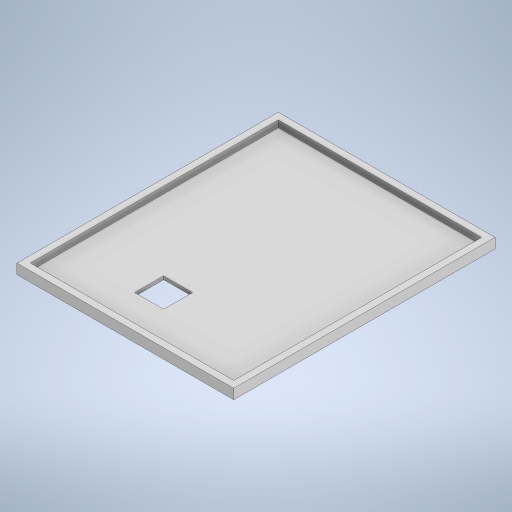
# Autodesk Inventor part: Tampa
Saved by Autodesk Inventor 2024 (Build 280153000, 153)
## iProperties
Created: 2023-09-01
Part Number: Tampa
Material: Genérico
Document SubType Name: Modeling
Designer: barof
Density: 1 g/cm^3
Appearance: Padrão
Author: barof
## iProperties of the stored document Tampa_3DPrint.ipt
Created: 2023-09-01
Part Number: Tampa_3DPrint
Material: Genérico
Document SubType Name: Modeling
Designer: barof
Density: 1 g/cm^3
Appearance: Padrão
Author: barof
Autodesk Inventor part; units mm, degrees
ref_plane "YZ Plane" through (0, 0, 0) normal (1, 0, 0) x (0, 1, 0)
ref_plane "XZ Plane" through (0, 0, 0) normal (0, 1, 0) x (-1, 0, 0)
ref_plane "XY Plane" through (0, 0, 0) normal (0, 0, 1) x (1, 0, 0)
sketch "Esboço1" plane through (0, 0, 0) normal (0, 1, 0) x (-1, 0, 0)
  line L0 (0, 0) -> (-97.4, 0)
  line L1 (-97.4, 0) -> (-97.4, -117.4)
  line L2 (-97.4, -117.4) -> (0, -117.4)
  line L3 (0, -117.4) -> (0, 0)
  line L4 (-3, -3) -> (-94.4, -3)
  line L5 (-94.4, -3) -> (-94.4, -114.4)
  line L6 (-94.4, -114.4) -> (-3, -114.4)
  line L7 (-3, -114.4) -> (-3, -3)
  point P0 (-48.7, -114.4)
  point P1 (-48.7, 0)
  point P2 (-48.7, -3)
  dimension "d2" = 3
  dimension "d3" = 3
  dimension "d4" = 3
  dimension "d5" = 3
  dimension "d6" = 91.4
  dimension "d7" = 111.4
  constraints: 16 end point, 4 parallel, 3 midpoint, 2 horizontal, 2 perpendicular
  measures "d2" distance from line of L2 point (-48.7, -114.4)
  measures "d3" distance between parallel lines of L1 L5
  measures "d4" distance between parallel lines of L3 L7
  measures "d5" distance of point (-48.7, 0) point (-48.7, -3)
  measures "d6" distance of L5.end L6.end
  measures "d7" distance of L4.end L5.end
extrude "Extrusão1" add sketch "Esboço1" along normal blind 1.5 contours L7 L6 L5 L4
extrude "Extrusão2" add sketch "Esboço1" along normal blind 4.5
sketch "Esboço2" plane through (0, 0, 0) normal (0, -1, 0) x (1, 0, 0)
  line L0 (47.925, -30.975) -> (34.925, -30.975)
  line L1 (34.925, -30.975) -> (34.925, -17.975)
  line L2 (34.925, -17.975) -> (47.925, -17.975)
  line L3 (47.925, -17.975) -> (47.925, -30.975)
  line L4 (0, 0) -> (97.4, 0) projected
  line L5 (0, -117.4) -> (0, 0) projected
  dimension "d12" = 13
  dimension "d13" = 13
  dimension "d16" = 17.975
  dimension "d17" = 34.925
  constraints: 8 end point, 2 parallel, 1 horizontal, 1 perpendicular
  measures "d12" distance of L1.end L2.end
  measures "d13" distance of L0.end L1.end
  measures "d16" distance between parallel lines of L4 L2
  measures "d17" distance between parallel lines of L5 L1
extrude "Extrusão3" cut sketch "Esboço2" against normal blind 10
